Autodesk Inventor part; units mm, degrees
(part 2 of 2)
  line L319 (-28.6263, 18.3241) -> (-28.6263, 16.0044)
  line L320 (-28.6263, 16.0044) -> (-25.6449, 16.0044)
  line L321 (-25.6449, 18.3241) -> (-28.6263, 18.3241)
  line L322 (-29.7503, 19.4482) -> (-24.5209, 19.4482)
  line L323 (-29.5884, 13.8513) -> (-27.9357, 13.8513)
  line L324 (-29.5884, 12.8808) -> (-29.5884, 13.8513)
  line L325 (-29.7503, 14.8804) -> (-29.7503, 19.4482)
  line L326 (-26.6942, 13.8513) -> (-19.7097, 13.8513)
  line L327 (-23.8, 11.9101) -> (-23.8, 12.8808)
  line L328 (-25.8364, 11.9101) -> (-23.8, 11.9101)
  line L329 (-24.7124, 10.786) -> (-24.7124, 8.4664)
  line L330 (-21.731, 8.4664) -> (-21.731, 10.786)
  line L331 (-24.7124, 8.4664) -> (-21.731, 8.4664)
  line L332 (-21.731, 10.786) -> (-24.7124, 10.786)
  line L333 (-26.6942, 14.8804) -> (-26.6942, 13.8513)
  line L334 (-24.5209, 14.8804) -> (-26.6942, 14.8804)
  line L335 (-20.607, 11.9101) -> (-20.607, 7.3423)
  line L336 (-20.607, 7.3423) -> (-25.8364, 7.3423)
  line L337 (-25.8364, 7.3423) -> (-25.8364, 11.9101)
  line L338 (-27.9357, 14.8804) -> (-29.7503, 14.8804)
  line L339 (-40.5846, 75.534) -> (-22.9154, 13.366) construction
  line L340 (-40.5846, 13.366) -> (-22.9154, 75.534) construction
  line L341 (-29.0204, 41.8116) -> (-29.0204, 39.4919)
  line L342 (-33.0307, 38.3371) -> (-38.2601, 38.3371)
  line L343 (-37.1361, 39.4611) -> (-34.1547, 39.4611)
  line L344 (-34.1547, 39.4611) -> (-34.1547, 41.7808)
  line L345 (-30.8654, 44.9353) -> (-25.077, 44.9353)
  line L346 (-34.9556, 42.9049) -> (-33.0307, 42.9049)
  line L347 (-34.1547, 41.7808) -> (-37.1361, 41.7808)
  line L348 (-38.9793, 44.9353) -> (-32.0432, 44.9353)
  line L349 (-34.9556, 43.9647) -> (-34.9556, 42.9049)
  line L350 (-36.0387, 42.9049) -> (-36.0387, 43.9647)
  line L351 (-38.2601, 42.9049) -> (-36.0387, 42.9049)
  line L352 (-36.0387, 43.9647) -> (-38.9793, 43.9647)
  line L353 (-37.1361, 41.7808) -> (-37.1361, 39.4611)
  line L354 (-38.2601, 38.3371) -> (-38.2601, 42.9049)
  line L355 (-26.7296, 43.9647) -> (-26.7296, 42.9356)
  line L356 (-32.0432, 44.9353) -> (-32.0432, 45.906)
  line L357 (-33.0307, 42.9049) -> (-33.0307, 38.3371)
  line L358 (-32.0432, 45.906) -> (-34.0584, 45.906)
  line L359 (-38.9793, 43.9647) -> (-38.9793, 44.9353)
  line L360 (-30.1445, 38.3679) -> (-30.1445, 42.9356)
  line L361 (-26.0391, 39.4919) -> (-26.0391, 41.8116)
  line L362 (-26.0391, 41.8116) -> (-29.0204, 41.8116)
  line L363 (-29.0204, 39.4919) -> (-26.0391, 39.4919)
  line L364 (-24.915, 38.3679) -> (-30.1445, 38.3679)
  line L365 (-25.077, 43.9647) -> (-26.7296, 43.9647)
  line L366 (-25.077, 44.9353) -> (-25.077, 43.9647)
  line L367 (-24.915, 42.9356) -> (-24.915, 38.3679)
  line L368 (-27.9712, 43.9647) -> (-34.9556, 43.9647)
  line L369 (-30.8654, 45.906) -> (-30.8654, 44.9353)
  line L370 (-28.829, 45.906) -> (-30.8654, 45.906)
  line L371 (-29.953, 47.03) -> (-29.953, 49.3497)
  line L372 (-32.9344, 49.3497) -> (-32.9344, 47.03)
  line L373 (-29.953, 49.3497) -> (-32.9344, 49.3497)
  line L374 (-32.9344, 47.03) -> (-29.953, 47.03)
  line L375 (-27.9712, 42.9356) -> (-27.9712, 43.9647)
  line L376 (-30.1445, 42.9356) -> (-27.9712, 42.9356)
  line L377 (-34.0584, 45.906) -> (-34.0584, 50.4737)
  line L378 (-34.0584, 50.4737) -> (-28.829, 50.4737)
  line L379 (-28.829, 50.4737) -> (-28.829, 45.906)
  line L380 (-26.7296, 42.9356) -> (-24.915, 42.9356)
  spline S0 degree 2 poles (-50.6582, 78.6307) (-50.6582, 77.8979) (-51.1275, 76.6465) (-51.5557, 76.1854) knots 0 0 0 1 2 2 2
  spline S1 degree 2 poles (-51.5557, 76.1854) (-51.9838, 75.7243) (-53.26, 75.1891) (-54.0504, 75.1891) knots 0 0 0 1 2 2 2
  spline S2 degree 2 poles (-54.0504, 75.1891) (-54.7749, 75.1891) (-56.1911, 75.5102) (-56.7098, 75.7655) knots 0 0 0 1 2 2 2
  line L381 (-56.7098, 75.7655) -> (-56.7098, 77.2063)
  line L382 (-56.7098, 77.2063) -> (-56.611, 77.2063)
  spline S3 degree 2 poles (-56.611, 77.2063) (-56.4545, 77.0911) (-55.87, 76.7947) (-55.5159, 76.6629) knots 0 0 0 1 2 2 2
  spline S4 degree 2 poles (-55.5159, 76.6629) (-55.1125, 76.523) (-54.4456, 76.3665) (-54.0257, 76.3665) knots 0 0 0 1 2 2 2
  spline S5 degree 2 poles (-54.0257, 76.3665) (-53.614, 76.3665) (-52.8401, 76.6629) (-52.5601, 76.984) knots 0 0 0 1 2 2 2
  spline S6 degree 2 poles (-52.5601, 76.984) (-52.3049, 77.2887) (-52.0414, 78.0955) (-52.0414, 78.6389) knots 0 0 0 1 2 2 2
  spline S7 degree 2 poles (-52.0414, 78.6389) (-52.0414, 79.1823) (-52.3378, 79.8739) (-52.6178, 80.1045) knots 0 0 0 1 2 2 2
  spline S8 degree 2 poles (-52.6178, 80.1045) (-52.9059, 80.3597) (-53.7622, 80.5738) (-54.2809, 80.5738) knots 0 0 0 1 2 2 2
  spline S9 degree 2 poles (-54.2809, 80.5738) (-54.8408, 80.5738) (-55.9523, 80.4009) (-56.2899, 80.3268) knots 0 0 0 1 2 2 2
  line L383 (-56.2899, 80.3268) -> (-56.2899, 85.5632)
  line L384 (-56.2899, 85.5632) -> (-50.7159, 85.5632)
  line L385 (-50.7159, 85.5632) -> (-50.7159, 84.3694)
  line L386 (-50.7159, 84.3694) -> (-54.9808, 84.3694)
  line L387 (-54.9808, 84.3694) -> (-54.9808, 81.6606)
  spline S10 degree 2 poles (-54.9808, 81.6606) (-54.7338, 81.6935) (-54.2562, 81.7182) (-54.0586, 81.7182) knots 0 0 0 1 2 2 2
  spline S11 degree 2 poles (-54.0586, 81.7182) (-53.2764, 81.7182) (-52.1979, 81.463) (-51.7039, 81.0842) knots 0 0 0 1 2 2 2
  spline S12 degree 2 poles (-51.7039, 81.0842) (-51.2016, 80.7055) (-50.6582, 79.5528) (-50.6582, 78.6307) knots 0 0 0 1 2 2 2
  spline S13 degree 2 poles (-12.8418, 10.4389) (-12.8418, 11.1717) (-12.3725, 12.4232) (-11.9443, 12.8843) knots 0 0 0 1 2 2 2
  spline S14 degree 2 poles (-11.9443, 12.8843) (-11.5162, 13.3453) (-10.24, 13.8805) (-9.4496, 13.8805) knots 0 0 0 1 2 2 2
  spline S15 degree 2 poles (-9.4496, 13.8805) (-8.7251, 13.8805) (-7.3089, 13.5594) (-6.7902, 13.3042) knots 0 0 0 1 2 2 2
  line L388 (-6.7902, 13.3042) -> (-6.7902, 11.8633)
  line L389 (-6.7902, 11.8633) -> (-6.889, 11.8633)
  spline S16 degree 2 poles (-6.889, 11.8633) (-7.0455, 11.9786) (-7.63, 12.275) (-7.9841, 12.4067) knots 0 0 0 1 2 2 2
  spline S17 degree 2 poles (-7.9841, 12.4067) (-8.3875, 12.5467) (-9.0544, 12.7031) (-9.4743, 12.7031) knots 0 0 0 1 2 2 2
  spline S18 degree 2 poles (-9.4743, 12.7031) (-9.886, 12.7031) (-10.6599, 12.4067) (-10.9399, 12.0856) knots 0 0 0 1 2 2 2
  spline S19 degree 2 poles (-10.9399, 12.0856) (-11.1951, 11.781) (-11.4586, 10.9741) (-11.4586, 10.4307) knots 0 0 0 1 2 2 2
  spline S20 degree 2 poles (-11.4586, 10.4307) (-11.4586, 9.8873) (-11.1622, 9.1957) (-10.8822, 8.9652) knots 0 0 0 1 2 2 2
  spline S21 degree 2 poles (-10.8822, 8.9652) (-10.5941, 8.7099) (-9.7378, 8.4959) (-9.2191, 8.4959) knots 0 0 0 1 2 2 2
  spline S22 degree 2 poles (-9.2191, 8.4959) (-8.6592, 8.4959) (-7.5477, 8.6688) (-7.2101, 8.7429) knots 0 0 0 1 2 2 2
  line L390 (-7.2101, 8.7429) -> (-7.2101, 3.5064)
  line L391 (-7.2101, 3.5064) -> (-12.7841, 3.5064)
  line L392 (-12.7841, 3.5064) -> (-12.7841, 4.7003)
  line L393 (-12.7841, 4.7003) -> (-8.5192, 4.7003)
  line L394 (-8.5192, 4.7003) -> (-8.5192, 7.4091)
  spline S23 degree 2 poles (-8.5192, 7.4091) (-8.7662, 7.3761) (-9.2438, 7.3514) (-9.4414, 7.3514) knots 0 0 0 1 2 2 2
  spline S24 degree 2 poles (-9.4414, 7.3514) (-10.2236, 7.3514) (-11.3021, 7.6067) (-11.7961, 7.9854) knots 0 0 0 1 2 2 2
  spline S25 degree 2 poles (-11.7961, 7.9854) (-12.2984, 8.3641) (-12.8418, 9.5168) (-12.8418, 10.4389) knots 0 0 0 1 2 2 2
  spline S26 degree 2 poles (-12.8418, 10.4389) (-12.8418, 11.1717) (-12.3725, 12.4232) (-11.9443, 12.8843) knots 0 0 0 1 2 2 2
  spline S27 degree 2 poles (-11.9443, 12.8843) (-11.5162, 13.3453) (-10.24, 13.8805) (-9.4496, 13.8805) knots 0 0 0 1 2 2 2
  spline S28 degree 2 poles (-9.4496, 13.8805) (-8.7251, 13.8805) (-7.3089, 13.5594) (-6.7902, 13.3042) knots 0 0 0 1 2 2 2
  line L395 (-6.7902, 13.3042) -> (-6.7902, 11.8633)
  line L396 (-6.7902, 11.8633) -> (-6.889, 11.8633)
  spline S29 degree 2 poles (-6.889, 11.8633) (-7.0455, 11.9786) (-7.63, 12.275) (-7.9841, 12.4067) knots 0 0 0 1 2 2 2
  spline S30 degree 2 poles (-7.9841, 12.4067) (-8.3875, 12.5467) (-9.0544, 12.7031) (-9.4743, 12.7031) knots 0 0 0 1 2 2 2
  spline S31 degree 2 poles (-9.4743, 12.7031) (-9.886, 12.7031) (-10.6599, 12.4067) (-10.9399, 12.0856) knots 0 0 0 1 2 2 2
  spline S32 degree 2 poles (-10.9399, 12.0856) (-11.1951, 11.781) (-11.4586, 10.9741) (-11.4586, 10.4307) knots 0 0 0 1 2 2 2
  spline S33 degree 2 poles (-11.4586, 10.4307) (-11.4586, 9.8873) (-11.1622, 9.1957) (-10.8822, 8.9652) knots 0 0 0 1 2 2 2
  spline S34 degree 2 poles (-10.8822, 8.9652) (-10.5941, 8.7099) (-9.7378, 8.4959) (-9.2191, 8.4959) knots 0 0 0 1 2 2 2
  spline S35 degree 2 poles (-9.2191, 8.4959) (-8.6592, 8.4959) (-7.5477, 8.6688) (-7.2101, 8.7429) knots 0 0 0 1 2 2 2
  line L397 (-7.2101, 8.7429) -> (-7.2101, 3.5064)
  line L398 (-7.2101, 3.5064) -> (-12.7841, 3.5064)
  line L399 (-12.7841, 3.5064) -> (-12.7841, 4.7003)
  line L400 (-12.7841, 4.7003) -> (-8.5192, 4.7003)
  line L401 (-8.5192, 4.7003) -> (-8.5192, 7.4091)
  spline S36 degree 2 poles (-8.5192, 7.4091) (-8.7662, 7.3761) (-9.2438, 7.3514) (-9.4414, 7.3514) knots 0 0 0 1 2 2 2
  spline S37 degree 2 poles (-9.4414, 7.3514) (-10.2236, 7.3514) (-11.3021, 7.6067) (-11.7961, 7.9854) knots 0 0 0 1 2 2 2
  spline S38 degree 2 poles (-11.7961, 7.9854) (-12.2984, 8.3641) (-12.8418, 9.5168) (-12.8418, 10.4389) knots 0 0 0 1 2 2 2
  spline S39 degree 2 poles (-50.6582, 78.6307) (-50.6582, 77.8979) (-51.1275, 76.6465) (-51.5557, 76.1854) knots 0 0 0 1 2 2 2
  spline S40 degree 2 poles (-51.5557, 76.1854) (-51.9838, 75.7243) (-53.26, 75.1891) (-54.0504, 75.1891) knots 0 0 0 1 2 2 2
  spline S41 degree 2 poles (-54.0504, 75.1891) (-54.7749, 75.1891) (-56.1911, 75.5102) (-56.7098, 75.7655) knots 0 0 0 1 2 2 2
  line L402 (-56.7098, 75.7655) -> (-56.7098, 77.2063)
  line L403 (-56.7098, 77.2063) -> (-56.611, 77.2063)
  spline S42 degree 2 poles (-56.611, 77.2063) (-56.4545, 77.0911) (-55.87, 76.7947) (-55.5159, 76.6629) knots 0 0 0 1 2 2 2
  spline S43 degree 2 poles (-55.5159, 76.6629) (-55.1125, 76.523) (-54.4456, 76.3665) (-54.0257, 76.3665) knots 0 0 0 1 2 2 2
  spline S44 degree 2 poles (-54.0257, 76.3665) (-53.614, 76.3665) (-52.8401, 76.6629) (-52.5601, 76.984) knots 0 0 0 1 2 2 2
  spline S45 degree 2 poles (-52.5601, 76.984) (-52.3049, 77.2887) (-52.0414, 78.0955) (-52.0414, 78.6389) knots 0 0 0 1 2 2 2
  spline S46 degree 2 poles (-52.0414, 78.6389) (-52.0414, 79.1823) (-52.3378, 79.8739) (-52.6178, 80.1045) knots 0 0 0 1 2 2 2
  spline S47 degree 2 poles (-52.6178, 80.1045) (-52.9059, 80.3597) (-53.7622, 80.5738) (-54.2809, 80.5738) knots 0 0 0 1 2 2 2
  spline S48 degree 2 poles (-54.2809, 80.5738) (-54.8408, 80.5738) (-55.9523, 80.4009) (-56.2899, 80.3268) knots 0 0 0 1 2 2 2
  line L404 (-56.2899, 80.3268) -> (-56.2899, 85.5632)
  line L405 (-56.2899, 85.5632) -> (-50.7159, 85.5632)
  line L406 (-50.7159, 85.5632) -> (-50.7159, 84.3694)
  line L407 (-50.7159, 84.3694) -> (-54.9808, 84.3694)
  line L408 (-54.9808, 84.3694) -> (-54.9808, 81.6606)
  spline S49 degree 2 poles (-54.9808, 81.6606) (-54.7338, 81.6935) (-54.2562, 81.7182) (-54.0586, 81.7182) knots 0 0 0 1 2 2 2
  spline S50 degree 2 poles (-54.0586, 81.7182) (-53.2764, 81.7182) (-52.1979, 81.463) (-51.7039, 81.0842) knots 0 0 0 1 2 2 2
  spline S51 degree 2 poles (-51.7039, 81.0842) (-51.2016, 80.7055) (-50.6582, 79.5528) (-50.6582, 78.6307) knots 0 0 0 1 2 2 2
  point P0 (-53.7479, 68.8958)
  point P1 (-9.7521, 20.0042)
  point P2 (-41.8348, 101.4209)
  point P3 (-53.7479, 68.8958)
  point P4 (-9.7521, 20.0042)
  point P5 (-1, 6.9835)
  point P6 (-94.7005, 61.8998)
  point P7 (-94.7005, 61.8998)
  point P8 (-31.75, 44.45)
  point P9 (-31.75, 44.45)
  dimension "d155" = 8.4153
  dimension "d157" = 0.508
  dimension "d158" = 4.5466
  dimension "d159" = 0.508
  dimension "d160" = 4.5466
  constraints: 736 end point, 50 parallel, 20 perpendicular, 14 horizontal, 5 midpoint, 1 symmetric about line, 14 other
  measures "d155" distance of L174.end L172.start
  measures "d157" distance between parallel lines of L7 L173
  measures "d158" distance from line of point (-1, 6.983) L172
  measures "d159" distance between parallel lines of L6 L168
  measures "d160" distance between parallel lines of L4 L171
extrude "Extrusion20" add sketch "Sketch17" along normal blind 0.4 contours L48 L49 L73 L71 L76 L69 L86 L79 L85 L67 L62 L68 L84 L80 L87 L77 L82 L60 L55 L61 L81 L78 L83 L70 L75 L72 L74 L50 | L88 L89 L113 L111 L116 L109 L126 L119 L125 L107 L102 L108 L124 L120 L127 L117 L122 L100 L95 L101 L121 L118 L123 L110 L115 L112 L114 L90 | L128 L129 L153 L151 L156 L149 L166 L159 L165 L147 L142 L148 L164 L160 L167 L157 L162 L140 L135 L141 L161 L158 L163 L150 L155 L152 L154 L130 | L219 L225 L226 L229 L230 L231 L234 L232 L233 L249 L247 L248 L257 L256 L237 L238 L239 L235 L246 L245 L244 L241 L255 L254 L258 L228 L223 L224 | L260 L272 L269 L268 L270 L277 L266 L274 L276 L295 L296 L297 L288 L287 L263 L284 L283 L273 L298 L285 L282 L278 L294 L293 L286 L267 L264 L275 | L300 L312 L309 L308 L310 L317 L306 L314 L316 L335 L336 L337 L328 L327 L303 L324 L323 L313 L338 L325 L322 L318 L334 L333 L326 L307 L304 L315 | L342 L354 L351 L350 L352 L359 L348 L356 L358 L377 L378 L379 L370 L369 L345 L366 L365 L355 L380 L367 L364 L360 L376 L375 L368 L349 L346 L357 | S0 S1 S2 L381 L382 S3 S4 S5 S6 S7 S8 S9 L383 L384 L385 L386 L387 S10 S11 S12 | S13 S14 S15 L388 L389 S16 S17 S18 S19 S20 S21 S22 L390 L391 L392 L393 L394 S23 S24 S25 bodies 2
sketch "Sketch18" plane through (0, 0, -0.2) normal (0, 0, -1) x (-1, 0, 0)
  line L0 (0, 0) -> (-63.5, 0)
  line L1 (-63.5, 0) -> (-63.5, 88.9)
  line L2 (-63.5, 88.9) -> (0, 88.9)
  line L3 (0, 88.9) -> (0, 0)
  constraints: 8 end point, 2 parallel, 1 horizontal, 1 perpendicular
extrude "Extrusion21" add sketch "Sketch18" along normal blind 0.4 bodies 3
fillet "Fillet2" radius 3.175 8 edges at (63.5, 0, 0.2) (63.5, 88.9, 0.2) (0, 0, 0.2) (0, 88.9, 0.2) (63.5, 0, -0.3) (63.5, 88.9, -0.3) (0, 0, -0.3) (0, 88.9, -0.3)
extrude "Extrusion22" cut sketch "Sketch17" along normal blind 0.4 contours L48 L49 L73 L71 L76 L69 L86 L79 L85 L67 L62 L68 L84 L80 L87 L77 L82 L60 L55 L61 L81 L78 L83 L70 L75 L72 L74 L50 | L88 L89 L113 L111 L116 L109 L126 L119 L125 L107 L102 L108 L124 L120 L127 L117 L122 L100 L95 L101 L121 L118 L123 L110 L115 L112 L114 L90 | L128 L129 L153 L151 L156 L149 L166 L159 L165 L147 L142 L148 L164 L160 L167 L157 L162 L140 L135 L141 L161 L158 L163 L150 L155 L152 L154 L130 | L219 L225 L226 L229 L230 L231 L234 L232 L233 L249 L247 L248 L257 L256 L237 L238 L239 L235 L246 L245 L244 L241 L255 L254 L258 L228 L223 L224 | L260 L272 L269 L268 L270 L277 L266 L274 L276 L295 L296 L297 L288 L287 L263 L284 L283 L273 L298 L285 L282 L278 L294 L293 L286 L267 L264 L275 | L300 L312 L309 L308 L310 L317 L306 L314 L316 L335 L336 L337 L328 L327 L303 L324 L323 L313 L338 L325 L322 L318 L334 L333 L326 L307 L304 L315 | L342 L354 L351 L350 L352 L359 L348 L356 L358 L377 L378 L379 L370 L369 L345 L366 L365 L355 L380 L367 L364 L360 L376 L375 L368 L349 L346 L357 | S0 S1 S2 L381 L382 S3 S4 S5 S6 S7 S8 S9 L383 L384 L385 L386 L387 S10 S11 S12 | S13 S14 S15 L388 L389 S16 S17 S18 S19 S20 S21 S22 L390 L391 L392 L393 L394 S23 S24 S25 bodies 3
